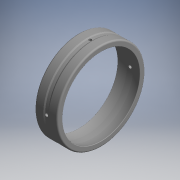
# Autodesk Inventor part: 21308 E_or
Saved by Autodesk Inventor 2017.3 (Build 213256000, 256)
## iProperties
Part Number: 21308 E_or
Material: Generic
Catalog Web Link: www.cadenas.de
Description: BS2_001-Spherical roller bearings
Vendor: SKF
Document SubType Name: Modeling
Designer: partserver
Manufacturer: SKF
Mass: 26.3855 g
Surface Area: 149.765 cm^2
Volume: 26.3855 cm^3
Density: 1 g/cm^3
Appearance: PSOLRGB-175-175-175
Category: PARTsolutions
Company: SKF
Title: 21308 E_or
Author: Cadenas PARTsolutions
Comments: Spherical roller bearings
PSOL_IDENT_0: {$CADENAS_DATA\23d-libs\skf\bearings_units_and_housings\roller_bearings\spherical_roller_bearings\pa
PSOL_IDENT_1: rts\bs2_001_or.prj},165 {VTYP=3D},{NB=21308 E_or},{LINA=21308 E_or},{NN=BS2_001},{DATE=23.12.2020 11
PSOL_IDENT_2: :58:30},{GEOMDATE=24.11.2020 12:50:21},{VERSION=},{LINEID=461840},{WBVAR=},{WBNUMERIC=}  {NB=21308 E
PSOL_IDENT_3: _or},{LINA=21308 E_or},{KT=DUMMY},{DESIGNATION=21308 E},{VARIANT=CE1W33},{DESIGNX=Cylindrical bore},
PSOL_IDENT_4: {SEAL=No seals},{SALG=NO},{BORE=40.000},{DD=40.000},{DD1=MIN},{D=90.000},{B=23.000},{DD2=60.000},{DD
PSOL_IDENT_5: 3=MIN},{D1=79.800},{B1=MIN},{B2=MIN},{B4=MIN},{B5=MIN},{BB=5.500},{K=3.000},{R12=1.500},{G=},{G1=MIN
PSOL_IDENT_6: },{TB=MIN},{ALPHA=9.0833},{R34=MIN},{PITCH=71.097},{DW=10.200},{LW=8.400},{DDAMIN=49.000},{DDAMAX=MI
PSOL_IDENT_7: N},{DBMIN=MIN},{DAMAX=81.000},{BAMIN=MIN},{RAMAX=1.500},{LOAD1=107.000},{LOAD2=108.000},{LOAD3=11.80
PSOL_IDENT_8: 0},{SPEED1=7000},{SPEED2=9500},{PRA=},{PLA=},{Z=19.000},{II=2.000},{MASS=0.740},{MASS2=MIN},{SLEEVE=
PSOL_IDENT_9: },{POPULAR=Yes},{BEARING=21308 E},{PPATH=parts/bs2_001_asmtpl.prj},{RAMAXX=1.5},{EE=0.24},{Y0=2.8},{
PSOL_IDENT_10: R12X=1.5},{Y2=4.2},{ALPHAX=9.08333},{Y1=2.8},{DD1X=},{B1X=},{SLEEVEX=},{ALPHAXX=},{B2X=},{SUPRESSED=
PSOL_IDENT_11: },{BBALG=5.500},{KALG=3.000},{Y=0.000}
NB: 21308 E_or
NN: BS2_001
NT: Spherical roller bearings
NBSYN: $DESIGNATION._or
LINA: 21308 E_or
CATALOG: SKF
DESIGNATION: 21308 E
VARIANT: CE1W33
DESIGNX: Cylindrical bore
SEAL: No seals
BORE: 40
DD: 40
DD1: 0
D: 90
B: 23
DD2: 60
DD3: 0
D1: 79.8
B1: 0
B2: 0
B4: 0
B5: 0
BB: 5.5
K: 3
R12: 1.5
G1: 0
TB: 0
ALPHA: 9.0833
R34: 0
PITCH: 71.097
DW: 10.2
LW: 8.4
DDAMIN: 49
DDAMAX: 0
DBMIN: 0
DAMAX: 81
BAMIN: 0
RAMAX: 1.5
LOAD1: 107
LOAD2: 108
LOAD3: 11.8
SPEED1: 7000
SPEED2: 9500
Z: 19
II: 2
MASS: 0.74
MASS2: 0
POPULAR: Yes
BEARING: 21308 E
PPATH: parts/bs2_001_asmtpl.prj
RAMAXX: 1.5
EE: 0.24
Y0: 2.8
R12X: 1.5
Y2: 4.2
ALPHAX: 9.08333
Y1: 2.8
Y: 0
SUPPLIER: SKF
ARTICLENO: 21308 E_or
BOMINFO: 21308 E_or
CREATOR: CADENAS GmbH
Autodesk Inventor part; units mm, degrees
sketch "Sketch_5" plane through (0, 0, 0) normal (0, 0, 1) x (1, 0, 0)
  line L0 (23, 0) -> (-23, 0)
  arc A0 (0, 39.9706) -> (0.4754, 39.6093) centre (0.375, 39.9706) ccw
  arc A1 (8.4397, 40.9891) -> (0.4754, 39.6093) centre (11.3621, 0.4458) ccw
  arc A2 (14.5603, 40.9891) -> (8.4397, 40.9891) centre (11.5, -308.9975) ccw
  arc A3 (22.5246, 39.6093) -> (14.5603, 40.9891) centre (11.6379, 0.4458) ccw
  arc A4 (22.5246, 39.6093) -> (23, 39.9706) centre (22.625, 39.9706) ccw
  line L1 (23, 39.9706) -> (23, 43.5)
  arc A5 (23, 43.5) -> (21.5, 45) centre (21.5, 43.5) ccw
  line L2 (21.5, 45) -> (14.25, 45)
  line L3 (14.25, 45) -> (13, 44.375)
  line L4 (13, 44.375) -> (10, 44.375)
  line L5 (10, 44.375) -> (8.75, 45)
  line L6 (8.75, 45) -> (1.5, 45)
  arc A6 (1.5, 45) -> (0, 43.5) centre (1.5, 43.5) ccw
  line L7 (0, 43.5) -> (0, 39.9706)
  constraints: 16 end point, 14 point on circle, 7 centre point
revolve "Revolution1" add sketch "Sketch_5" angle 360 about axis through (23, 0, 0) along (1, 0, 0)
sketch "Sketch_2" plane through (0, 0, 0) normal (0, 0, 1) x (1, 0, 0)
  line L0 (11.5, -45) -> (11.5, -39.9)
  line L1 (11.5, -39.9) -> (13, -39.9)
  line L2 (13, -39.9) -> (13, -45)
  line L3 (13, -45) -> (11.5, -45)
  line L4 (11.5, -45) -> (11.5, -39.9)
  constraints: 10 end point
revolve "Revolution2" cut sketch "Sketch_2" angle 360 about axis through (11.5, -45, 0) along (0, -1, 0)
sketch "Sketch_9" plane through (0, 0, 0) normal (0, 1, 0) x (-1, 0, 0)
  line L0 (-11.5, -39.9) -> (-11.5, -45)
  line L1 (-11.5, -45) -> (-13, -45)
  line L2 (-13, -45) -> (-13, -39.9)
  line L3 (-13, -39.9) -> (-11.5, -39.9)
  line L4 (-11.5, -39.9) -> (-11.5, -45)
  constraints: 10 end point
revolve "Revolution3" cut sketch "Sketch_9" angle 360 about axis through (11.5, 0, -39.9) along (0, 0, 1)
sketch "Sketch_10" plane through (0, 0, 0) normal (0, 0, 1) x (1, 0, 0)
  line L0 (11.5, 39.9) -> (11.5, 45)
  line L1 (11.5, 45) -> (13, 45)
  line L2 (13, 45) -> (13, 39.9)
  line L3 (13, 39.9) -> (11.5, 39.9)
  line L4 (11.5, 39.9) -> (11.5, 45)
  constraints: 10 end point
revolve "Revolution4" cut sketch "Sketch_10" angle 360 about axis through (11.5, 39.9, 0) along (0, -1, 0)
ref_plane "NO_GEO_XY" through (0, 0, 0) normal (1, 0, 0) x (0, 0, -1)
ref_plane "NO_GEO_YZ" through (0, 0, 0) normal (0, 0, -1) x (0, 1, 0)
ref_plane "NO_GEO_ZX" through (0, 0, 0) normal (0, 1, 0) x (1, 0, 0)
ref_plane "or_XY" through (0, 0, 0) normal (0, 0, 1) x (1, 0, 0)
ref_plane "or_YZ" through (0, 0, 0) normal (1, 0, 0) x (0, 1, 0)
ref_plane "or_ZX" through (0, 0, 0) normal (0, 1, 0) x (0, 0, 1)
body "Solid1"
